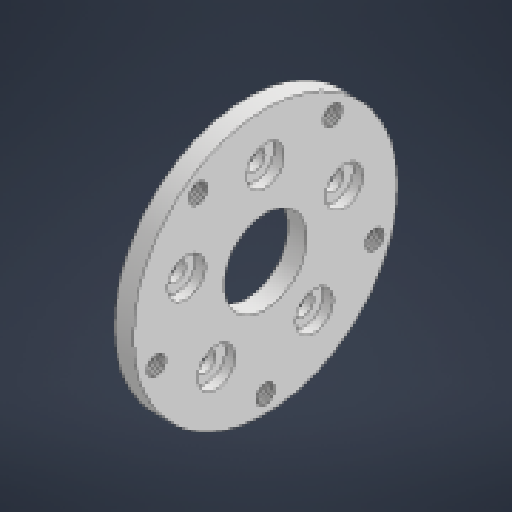
# Autodesk Inventor part: spacer_flange
Saved by Autodesk Inventor 2023.2 (Build 272271030, 271C)
## iProperties
Created: 2023-11-12
Part Number: spacer_flange
Material: Generic
Document SubType Name: Modeling
Designer: ralph
Density: 1 g/cm^3
Appearance: Default
Author: ralph
Autodesk Inventor part; units mm, degrees
ref_plane "YZ Plane" through (0, 0, 0) normal (1, 0, 0) x (0, 1, 0)
ref_plane "XZ Plane" through (0, 0, 0) normal (0, 1, 0) x (-1, 0, 0)
ref_plane "XY Plane" through (0, 0, 0) normal (0, 0, 1) x (1, 0, 0)
sketch "Sketch1" plane through (0, 0, 0) normal (1, 0, 0) x (0, 1, 0)
  circle A0 centre (0, 0) radius 13.97
  circle A1 centre (0, 0) radius 44.45
  dimension "d0" = 27.94
  dimension "d1" = 88.9
  constraints: 2 centre point, 2 coincident
  measures "d0" diameter of A0
  measures "d1" diameter of A1
extrude "Extrusion1" add sketch "Sketch1" along normal blind 6.35
sketch "Sketch2" plane through (6.35, 0, 0) normal (1, 0, 0) x (0, 0, -1)
  arc A0 (25.458, -0.8256) -> (35.4837, 5.2699) centre (26.5725, 8.6339) ccw projected
  arc A1 (25.6093, -25.1202) -> (21.0812, -14.2959) centre (16.4227, -22.6039) ccw projected
  arc A2 (37.0087, -36.5562) -> (51.4278, 7.8214) centre (0, 0) ccw projected
  circle A3 centre (36.7212, -11.9315) radius 13.4082
  circle A4 centre (36.7212, -11.9315) radius 3.175
  circle A5 centre (22.695, 31.237) radius 3.175
  circle A6 centre (-22.695, 31.237) radius 3.175
  circle A7 centre (-36.7212, -11.9315) radius 3.175
  circle A8 centre (0, -38.611) radius 3.175
  point P0 (0, 0)
  dimension "d4" = 6.35
  dimension "d7" = 360
  constraints: 6 centre point, 3 tangent, 1 coincident, 11 other
  measures "d4" diameter of A4
extrude "Extrusion2" cut sketch "Sketch2" against normal through all contours A4 | A5 | A6 | A7 | A8
thread "Thread1" size "1/4-20 UNC" class "2B" standard "ANSI Unified Screw Threads" full length
thread "Thread2" size "1/4-20 UNC" class "2B" standard "ANSI Unified Screw Threads" full length
thread "Thread3" size "1/4-20 UNC" class "2B" standard "ANSI Unified Screw Threads" full length
thread "Thread4" size "1/4-20 UNC" class "2B" standard "ANSI Unified Screw Threads" full length
thread "Thread5" size "1/4-20 UNC" class "2B" standard "ANSI Unified Screw Threads" full length
sketch "Sketch3" plane through (6.35, 0, 0) normal (1, 0, 0) x (0, 0, -1)
  circle A0 centre (26.5725, 8.6339) radius 1.27 projected
  circle A1 centre (26.5725, 8.6339) radius 3.175
  circle A2 centre (0, 27.94) radius 3.175
  circle A3 centre (-26.5725, 8.6339) radius 3.175
  circle A4 centre (-16.4227, -22.6039) radius 3.175
  circle A5 centre (16.4227, -22.6039) radius 3.175
  point P0 (0, 0)
  dimension "d21" = 6.35
  dimension "d24" = 360
  constraints: 5 centre point, 1 coincident, 11 other
  measures "d21" diameter of A1
extrude "Extrusion3" cut sketch "Sketch3" against normal up to next contours A0 | A1 | A2 | A3 | A4 | A5
sketch "Sketch4" plane through (6.35, 0, 0) normal (1, 0, 0) x (0, 0, -1)
  circle A0 centre (26.5725, 8.6339) radius 3.175 projected
  circle A1 centre (26.5725, 8.6339) radius 6.35
  circle A2 centre (0, 27.94) radius 6.35
  circle A3 centre (-26.5725, 8.6339) radius 6.35
  circle A4 centre (-16.4227, -22.6039) radius 6.35
  circle A5 centre (16.4227, -22.6039) radius 6.35
  point P0 (0, 0)
  dimension "d28" = 12.7
  dimension "d33" = 360
  constraints: 5 centre point, 1 coincident, 11 other
  measures "d28" diameter of A1
extrude "Extrusion4" cut sketch "Sketch4" against normal blind 3.429
body "Solid1"
